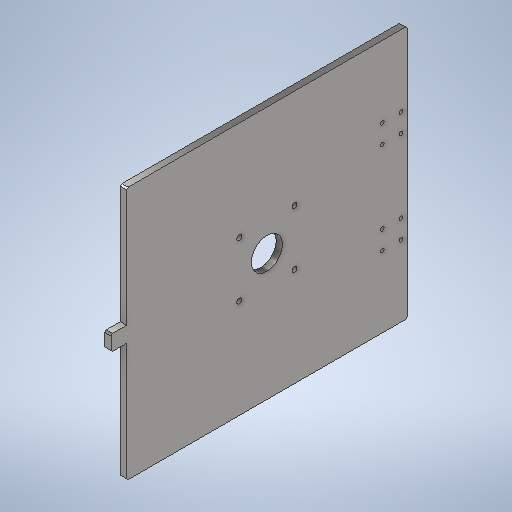
# Autodesk Inventor part: CTQCX300.2-1门板
Saved by Autodesk Inventor 2025.1 (Build 291241000, 241)
## iProperties
Created: 2025-06-20
Part Number: CTQCX300.2-1门板
Material: 钢板B-8/SUS304
Document SubType Name: Modeling
Designer: TengX
Density: 8 g/cm^3
Appearance: 半抛光
Mass: 4958.68 g
Surface Area: 1667.44 cm^2
Volume: 619.835 cm^3
Author: TengX
Autodesk Inventor part; units mm, degrees
ref_plane "YZ Plane" through (0, 0, 0) normal (1, 0, 0) x (0, 1, 0)
ref_plane "XZ Plane" through (0, 0, 0) normal (0, 1, 0) x (-1, 0, 0)
ref_plane "XY Plane" through (0, 0, 0) normal (0, 0, 1) x (1, 0, 0)
sketch "草图1" plane through (0, 0, 0) normal (1, 0, 0) x (0, 1, 0)
  line L0 (162.5, 180) -> (-162.5, 180)
  line L1 (-162.5, 180) -> (-162.5, -180)
  line L2 (-162.5, -180) -> (162.5, -180)
  line L3 (162.5, -180) -> (162.5, 180)
  line L4 (162.5, 180) -> (-162.5, -180) construction
  line L5 (-162.5, 180) -> (162.5, -180) construction
  circle A0 centre (0, 0) radius 20
  line L6 (-10, 200) -> (10, 200)
  line L7 (10, 200) -> (10, 180)
  line L8 (10, 180) -> (-10, 180)
  line L9 (-10, 180) -> (-10, 200)
  line L10 (-10, 200) -> (10, 180) construction
  line L11 (10, 200) -> (-10, 180) construction
  point P0 (0, 190)
  point P1 (0, 190)
  dimension "d0" = 325
  dimension "d1" = 360
  dimension "d2" = 40
  dimension "d54" = 20
  dimension "d55" = 20
  constraints: 24 end point, 5 midpoint, 5 parallel, 2 perpendicular, 1 centre point, 1 coincident, 1 horizontal, 1 point on line, 1 vertical alignment
  measures "d0" distance of L0.start L0.end
  measures "d1" distance of L2.end L0.start
  measures "d2" diameter of A0
  measures "d54" distance of L8.end L6.start
  measures "d55" distance of L6.start L6.end
extrude "拉伸1" add sketch "草图1" along normal blind 8
chamfer "倒角1" distance 2 angle 45 4 edges at (4, 162.5, 180) (4, 162.5, -180) (4, -162.5, 180) (4, -162.5, -180)
sketch "草图2" plane through (8, 0, 0) normal (1, 0, 0) x (0, 0, -1)
  line L0 (178, 162.5) -> (-178, 162.5) projected
  line L1 (-180, 160.5) -> (-180, -160.5) projected
  line L2 (180, -160.5) -> (180, 160.5) projected
  line L3 (-178, -162.5) -> (178, -162.5) projected
  point P0 (0, 0)
  point P1 (148, 71)
  point P2 (148, 47)
  point P3 (172, 71)
  point P4 (172, 47)
  point P5 (172, -71)
  point P6 (172, -47)
  point P7 (148, -71)
  point P8 (148, -47)
  dimension "d8" = 91.5
  dimension "d12" = 24
  dimension "d15" = 24
  dimension "d20" = 118
  dimension "d25" = 94
  dimension "d26" = 142
  dimension "d27" = 352
  dimension "d50" = 8
  dimension "d51" = 91.5
  constraints: 2 vertical, 1 horizontal, 7 other
  measures "d8" distance from line of L0 point (148, 71)
  measures "d12" distance of point (148, 71) point (148, 47)
  measures "d15" distance of point (148, 71) point (172, 71)
  measures "d20" distance of point (172, 47) point (172, -71)
  measures "d25" distance of point (148, -47) point (148, 47)
  measures "d26" distance of point (148, -71) point (148, 71)
  measures "d27" distance from line of L1 point (172, -71)
  measures "d50" distance from line of L2 point (172, 71)
  measures "d51" distance from line of L3 point (172, -71)
hole "孔1" at (8, 71, -148) at (8, 47, -148) at (8, 71, -172) at (8, 47, -172) at (8, -71, -172) at (8, -47, -172) at (8, -71, -148) at (8, -47, -148) direction (-1, 0, 0) diameter 4.917 end through all thread size "M6x1" designation "M6" class "6H" standard "GB Metric profile"
sketch "草图3" plane through (8, 0, 0) normal (1, 0, 0) x (0, 0, -1)
  line L0 (0, 0) -> (-35.3553, 35.3553) construction
  line L1 (-178, -162.5) -> (178, -162.5) projected
  line L2 (0, 0) -> (-35.3553, -35.3553) construction
  line L3 (0, 0) -> (35.3553, -35.3553) construction
  line L4 (0, 0) -> (35.3553, 35.3553) construction
  dimension "d35" = 45
  dimension "d36" = 50
  dimension "d39" = 360
  constraints: 8 end point, 6 coincident, 15 other
  measures "d35" angle of L1 L0
  measures "d36" distance of L0.start L0.end
hole "孔2" at (8, 35.3553, 35.3553) at (8, -35.3553, 35.3553) at (8, -35.3553, -35.3553) at (8, 35.3553, -35.3553) direction (-1, 0, 0) diameter 6.647 end through all thread size "M8x1.25" designation "M8" class "6H" standard "GB Metric profile"
chamfer "倒角2" distance 2 angle 45 2 edges at (4, 10, 200) (4, -10, 200)
